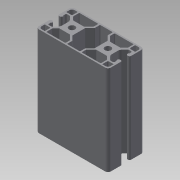
# Autodesk Inventor part: 40-4085-LITE
Saved by Autodesk Inventor 2013 (Build 170138000, 138)
## iProperties
Created: 2014-04-23
Part Number: 40-4085-LITE
Material: Generic
Document SubType Name: Modeling
Designer: Ross Bowman
Density: 1 g/cm^3
Engineer: Ross Bowman
Catalog Web Link: 8020.net
Vendor: 80/20 Inc.
Company: 80/20 Inc.
Author: Ross Bowman
Keywords: 80/20 , 8020 , T-Slot , Extrusion
Material: 6105-T5 Aluminum
Autodesk Inventor part; units mm, degrees
ref_plane "YZ Plane" through (0, 0, 0) normal (1, 0, 0) x (0, 1, 0)
ref_plane "XZ Plane" through (0, 0, 0) normal (0, 1, 0) x (-1, 0, 0)
ref_plane "XY Plane" through (0, 0, 0) normal (0, 0, 1) x (1, 0, 0)
sketch "Sketch1" plane through (0, 0, 0) normal (0, 0, 1) x (1, 0, 0)
  circle A0 centre (-20, 0) radius 3.3778
  circle A1 centre (20, 0) radius 3.3778
  arc A2 (-7.1746, -12.8345) -> (-7.435, -12.2058) centre (-8.0636, -12.8345) ccw
  line L0 (-12.0571, -7.5838) -> (-7.435, -12.2058)
  arc A3 (-12.3175, -6.9551) -> (-12.0571, -7.5838) centre (-11.4285, -6.9551) ccw
  line L1 (-12.3175, 7.0078) -> (-12.3175, -6.9551)
  arc A4 (-12.0943, 7.5465) -> (-12.3175, 7.0078) centre (-11.5556, 7.0078) ccw
  line L2 (-7.3343, 12.3066) -> (-12.0943, 7.5465)
  arc A5 (-7.3343, 12.3066) -> (-7.1111, 12.8453) centre (-7.873, 12.8453) ccw
  line L3 (-7.1111, 17.5873) -> (-7.1111, 12.8453)
  arc A6 (-6.3492, 18.3492) -> (-7.1111, 17.5873) centre (-6.3492, 17.5873) ccw
  line L4 (6.3492, 18.3492) -> (-6.3492, 18.3492)
  arc A7 (7.1111, 17.5873) -> (6.3492, 18.3492) centre (6.3492, 17.5873) ccw
  line L5 (7.1111, 12.8453) -> (7.1111, 17.5873)
  arc A8 (7.1111, 12.8453) -> (7.3343, 12.3066) centre (7.873, 12.8453) ccw
  line L6 (12.0943, 7.5465) -> (7.3343, 12.3066)
  arc A9 (12.3175, 7.0078) -> (12.0943, 7.5465) centre (11.5556, 7.0078) ccw
  line L7 (12.3175, -6.9551) -> (12.3175, 7.0078)
  arc A10 (12.0571, -7.5838) -> (12.3175, -6.9551) centre (11.4285, -6.9551) ccw
  line L8 (7.435, -12.2058) -> (12.0571, -7.5838)
  arc A11 (7.435, -12.2058) -> (7.1746, -12.8345) centre (8.0636, -12.8345) ccw
  line L9 (7.1746, -17.5873) -> (7.1746, -12.8345)
  arc A12 (6.4127, -18.3492) -> (7.1746, -17.5873) centre (6.4127, -17.5873) ccw
  line L10 (-6.4127, -18.3492) -> (6.4127, -18.3492)
  arc A13 (-7.1746, -17.5873) -> (-6.4127, -18.3492) centre (-6.4127, -17.5873) ccw
  line L11 (-7.1746, -12.8345) -> (-7.1746, -17.5873)
  arc A14 (9.239, -13.0955) -> (9.0159, -13.6343) centre (9.7778, -13.6343) ccw
  line L12 (14.4289, -7.9057) -> (9.239, -13.0955)
  arc A15 (14.9676, -7.6825) -> (14.4289, -7.9057) centre (14.9676, -8.4444) ccw
  line L13 (26.1099, -7.6825) -> (14.9676, -7.6825)
  arc A16 (26.6486, -7.9057) -> (26.1099, -7.6825) centre (26.1099, -8.4444) ccw
  line L14 (30.0626, -11.3196) -> (26.6486, -7.9057)
  arc A17 (30.2857, -11.8584) -> (30.0626, -11.3196) centre (29.5238, -11.8584) ccw
  line L15 (30.2857, -17.5873) -> (30.2857, -11.8584)
  arc A18 (29.5238, -18.3492) -> (30.2857, -17.5873) centre (29.5238, -17.5873) ccw
  line L16 (9.7778, -18.3492) -> (29.5238, -18.3492)
  arc A19 (9.0159, -17.5873) -> (9.7778, -18.3492) centre (9.7778, -17.5873) ccw
  line L17 (9.0159, -13.6343) -> (9.0159, -17.5873)
  arc A20 (-26.6486, 7.9057) -> (-26.1099, 7.6825) centre (-26.1099, 8.4444) ccw
  line L18 (-30.0626, 11.3196) -> (-26.6486, 7.9057)
  arc A21 (-30.2857, 11.8584) -> (-30.0626, 11.3196) centre (-29.5238, 11.8584) ccw
  line L19 (-30.2857, 17.5873) -> (-30.2857, 11.8584)
  arc A22 (-29.5238, 18.3492) -> (-30.2857, 17.5873) centre (-29.5238, 17.5873) ccw
  line L20 (-9.7778, 18.3492) -> (-29.5238, 18.3492)
  arc A23 (-9.0159, 17.5873) -> (-9.7778, 18.3492) centre (-9.7778, 17.5873) ccw
  line L21 (-9.0159, 13.6343) -> (-9.0159, 17.5873)
  arc A24 (-9.239, 13.0955) -> (-9.0159, 13.6343) centre (-9.7778, 13.6343) ccw
  line L22 (-14.4289, 7.9057) -> (-9.239, 13.0955)
  arc A25 (-14.9676, 7.6825) -> (-14.4289, 7.9057) centre (-14.9676, 8.4444) ccw
  line L23 (-26.1099, 7.6825) -> (-14.9676, 7.6825)
  arc A26 (-26.1099, -7.6825) -> (-26.6486, -7.9057) centre (-26.1099, -8.4444) ccw
  line L24 (-14.9676, -7.6825) -> (-26.1099, -7.6825)
  arc A27 (-14.4289, -7.9057) -> (-14.9676, -7.6825) centre (-14.9676, -8.4444) ccw
  line L25 (-9.239, -13.0955) -> (-14.4289, -7.9057)
  arc A28 (-9.0159, -13.6343) -> (-9.239, -13.0955) centre (-9.7778, -13.6343) ccw
  line L26 (-9.0159, -17.5873) -> (-9.0159, -13.6343)
  arc A29 (-9.7778, -18.3492) -> (-9.0159, -17.5873) centre (-9.7778, -17.5873) ccw
  line L27 (-29.5238, -18.3492) -> (-9.7778, -18.3492)
  arc A30 (-30.2857, -17.5873) -> (-29.5238, -18.3492) centre (-29.5238, -17.5873) ccw
  line L28 (-30.2857, -11.8584) -> (-30.2857, -17.5873)
  arc A31 (-30.0626, -11.3196) -> (-30.2857, -11.8584) centre (-29.5238, -11.8584) ccw
  line L29 (-26.6486, -7.9057) -> (-30.0626, -11.3196)
  arc A32 (9.7778, 18.3492) -> (9.0159, 17.5873) centre (9.7778, 17.5873) ccw
  line L30 (29.5238, 18.3492) -> (9.7778, 18.3492)
  arc A33 (30.2857, 17.5873) -> (29.5238, 18.3492) centre (29.5238, 17.5873) ccw
  line L31 (30.2857, 11.8584) -> (30.2857, 17.5873)
  arc A34 (30.0626, 11.3196) -> (30.2857, 11.8584) centre (29.5238, 11.8584) ccw
  line L32 (26.6486, 7.9057) -> (30.0626, 11.3196)
  arc A35 (26.1099, 7.6825) -> (26.6486, 7.9057) centre (26.1099, 8.4444) ccw
  line L33 (14.9676, 7.6825) -> (26.1099, 7.6825)
  arc A36 (14.4289, 7.9057) -> (14.9676, 7.6825) centre (14.9676, 8.4444) ccw
  line L34 (9.239, 13.0955) -> (14.4289, 7.9057)
  arc A37 (9.0159, 13.6343) -> (9.239, 13.0955) centre (9.7778, 13.6343) ccw
  line L35 (9.0159, 17.5873) -> (9.0159, 13.6343)
  arc A38 (32.3165, 18.3492) -> (31.9365, 17.9693) centre (32.3165, 17.9693) ccw
  line L36 (35.5555, 18.3492) -> (32.3165, 18.3492)
  arc A39 (38.3495, 15.5552) -> (35.5555, 18.3492) centre (35.5555, 15.5552) ccw
  line L37 (38.3495, 12.3165) -> (38.3495, 15.5552)
  arc A40 (37.9695, 11.9365) -> (38.3495, 12.3165) centre (37.9695, 12.3165) ccw
  line L38 (33.2063, 11.9365) -> (37.9695, 11.9365)
  arc A41 (31.9365, 13.2063) -> (33.2063, 11.9365) centre (33.2063, 13.2063) ccw
  line L39 (31.9365, 17.9693) -> (31.9365, 13.2063)
  arc A42 (35.5555, -18.3492) -> (38.3495, -15.5552) centre (35.5555, -15.5552) ccw
  line L40 (32.3165, -18.3492) -> (35.5555, -18.3492)
  arc A43 (31.9365, -17.9693) -> (32.3165, -18.3492) centre (32.3165, -17.9693) ccw
  line L41 (31.9365, -13.2063) -> (31.9365, -17.9693)
  arc A44 (33.2063, -11.9365) -> (31.9365, -13.2063) centre (33.2063, -13.2063) ccw
  line L42 (37.9695, -11.9365) -> (33.2063, -11.9365)
  arc A45 (38.3495, -12.3165) -> (37.9695, -11.9365) centre (37.9695, -12.3165) ccw
  line L43 (38.3495, -15.5552) -> (38.3495, -12.3165)
  arc A46 (-35.5555, 18.3492) -> (-38.3495, 15.5552) centre (-35.5555, 15.5552) ccw
  line L44 (-32.3165, 18.3492) -> (-35.5555, 18.3492)
  arc A47 (-31.9365, 17.9693) -> (-32.3165, 18.3492) centre (-32.3165, 17.9693) ccw
  line L45 (-31.9365, 13.2063) -> (-31.9365, 17.9693)
  arc A48 (-33.2063, 11.9365) -> (-31.9365, 13.2063) centre (-33.2063, 13.2063) ccw
  line L46 (-37.9695, 11.9365) -> (-33.2063, 11.9365)
  arc A49 (-38.3495, 12.3165) -> (-37.9695, 11.9365) centre (-37.9695, 12.3165) ccw
  line L47 (-38.3495, 15.5552) -> (-38.3495, 12.3165)
  arc A50 (-32.3165, -18.3492) -> (-31.9365, -17.9693) centre (-32.3165, -17.9693) ccw
  line L48 (-35.5555, -18.3492) -> (-32.3165, -18.3492)
  arc A51 (-38.3495, -15.5552) -> (-35.5555, -18.3492) centre (-35.5555, -15.5552) ccw
  line L49 (-38.3495, -12.3165) -> (-38.3495, -15.5552)
  arc A52 (-37.9695, -11.9365) -> (-38.3495, -12.3165) centre (-37.9695, -12.3165) ccw
  line L50 (-33.2063, -11.9365) -> (-37.9695, -11.9365)
  arc A53 (-31.9365, -13.2063) -> (-33.2063, -11.9365) centre (-33.2063, -13.2063) ccw
  line L51 (-31.9365, -17.9693) -> (-31.9365, -13.2063)
  arc A54 (35.4286, -10.2857) -> (36.6984, -9.0159) centre (35.4286, -9.0159) ccw
  line L52 (35.4286, -10.2857) -> (32.9885, -10.2857)
  arc A55 (32.3599, -10.0254) -> (32.9885, -10.2857) centre (32.9885, -9.3968) ccw
  line L53 (32.3599, -10.0254) -> (29.0736, -6.739)
  arc A56 (27.6825, -3.3808) -> (29.0736, -6.739) centre (32.4317, -3.3808) ccw
  line L54 (27.6825, -3.3808) -> (27.6825, 3.3808)
  arc A57 (29.0736, 6.739) -> (27.6825, 3.3808) centre (32.4317, 3.3808) ccw
  line L55 (29.0736, 6.739) -> (32.3599, 10.0254)
  arc A58 (32.9885, 10.2857) -> (32.3599, 10.0254) centre (32.9885, 9.3968) ccw
  line L56 (32.9885, 10.2857) -> (35.4286, 10.2857)
  arc A59 (36.6984, 9.0159) -> (35.4286, 10.2857) centre (35.4286, 9.0159) ccw
  line L57 (36.6984, 9.0159) -> (36.6984, 7.1685)
  arc A60 (36.3317, 6.7888) -> (36.6984, 7.1685) centre (36.3185, 7.1685) ccw
  line L58 (36.3317, 6.7888) -> (36.3032, 6.7878)
  arc A61 (36.3032, 6.7878) -> (35.9365, 6.4081) centre (36.3165, 6.4081) ccw
  line L59 (35.9365, 6.4081) -> (35.9365, 5.6381)
  arc A62 (35.9365, 5.6381) -> (37.5111, 4.0635) centre (37.5111, 5.6381) ccw
  line L60 (37.5111, 4.0635) -> (38.4254, 4.0635)
  arc A63 (38.4254, 4.0635) -> (40, 5.6381) centre (38.4254, 5.6381) ccw
  line L61 (40, 5.6381) -> (40, 16.8254)
  arc A64 (40, 16.8254) -> (36.8254, 20) centre (36.8254, 16.8254) ccw
  line L62 (36.8254, 20) -> (-36.8254, 20)
  arc A65 (-36.8254, 20) -> (-40, 16.8254) centre (-36.8254, 16.8254) ccw
  line L63 (-40, 16.8254) -> (-40, 5.6381)
  arc A66 (-40, 5.6381) -> (-38.4254, 4.0635) centre (-38.4254, 5.6381) ccw
  line L64 (-38.4254, 4.0635) -> (-37.5111, 4.0635)
  arc A67 (-37.5111, 4.0635) -> (-35.9365, 5.6381) centre (-37.5111, 5.6381) ccw
  line L65 (-35.9365, 5.6381) -> (-35.9365, 6.3446)
  arc A68 (-35.9365, 6.3446) -> (-36.3032, 6.7243) centre (-36.3165, 6.3446) ccw
  line L66 (-36.3032, 6.7243) -> (-36.3317, 6.7253)
  arc A69 (-36.6984, 7.105) -> (-36.3317, 6.7253) centre (-36.3185, 7.105) ccw
  line L67 (-36.6984, 7.105) -> (-36.6984, 9.0159)
  arc A70 (-35.4286, 10.2857) -> (-36.6984, 9.0159) centre (-35.4286, 9.0159) ccw
  line L68 (-35.4286, 10.2857) -> (-32.9885, 10.2857)
  arc A71 (-32.3599, 10.0254) -> (-32.9885, 10.2857) centre (-32.9885, 9.3968) ccw
  line L69 (-32.3599, 10.0254) -> (-29.0736, 6.739)
  arc A72 (-27.6825, 3.3808) -> (-29.0736, 6.739) centre (-32.4317, 3.3808) ccw
  line L70 (-27.6825, 3.3808) -> (-27.6825, -3.3808)
  arc A73 (-29.0736, -6.739) -> (-27.6825, -3.3808) centre (-32.4317, -3.3808) ccw
  line L71 (-29.0736, -6.739) -> (-32.3599, -10.0254)
  arc A74 (-32.9885, -10.2857) -> (-32.3599, -10.0254) centre (-32.9885, -9.3968) ccw
  line L72 (-32.9885, -10.2857) -> (-35.4286, -10.2857)
  arc A75 (-36.6984, -9.0159) -> (-35.4286, -10.2857) centre (-35.4286, -9.0159) ccw
  line L73 (-36.6984, -9.0159) -> (-36.6984, -7.105)
  arc A76 (-36.3317, -6.7253) -> (-36.6984, -7.105) centre (-36.3185, -7.105) ccw
  line L74 (-36.3317, -6.7253) -> (-36.3032, -6.7243)
  arc A77 (-36.3032, -6.7243) -> (-35.9365, -6.3446) centre (-36.3165, -6.3446) ccw
  line L75 (-35.9365, -6.3446) -> (-35.9365, -5.6381)
  arc A78 (-35.9365, -5.6381) -> (-37.5111, -4.0635) centre (-37.5111, -5.6381) ccw
  line L76 (-37.5111, -4.0635) -> (-38.4254, -4.0635)
  arc A79 (-38.4254, -4.0635) -> (-40, -5.6381) centre (-38.4254, -5.6381) ccw
  line L77 (-40, -5.6381) -> (-40, -16.8254)
  arc A80 (-40, -16.8254) -> (-36.8254, -20) centre (-36.8254, -16.8254) ccw
  line L78 (-36.8254, -20) -> (36.8254, -20)
  arc A81 (36.8254, -20) -> (40, -16.8254) centre (36.8254, -16.8254) ccw
  line L79 (40, -16.8254) -> (40, -5.6381)
  arc A82 (40, -5.6381) -> (38.4254, -4.0635) centre (38.4254, -5.6381) ccw
  line L80 (38.4254, -4.0635) -> (37.5111, -4.0635)
  arc A83 (37.5111, -4.0635) -> (35.9365, -5.6381) centre (37.5111, -5.6381) ccw
  line L81 (35.9365, -5.6381) -> (35.9365, -6.4081)
  arc A84 (35.9365, -6.4081) -> (36.3032, -6.7878) centre (36.3165, -6.4081) ccw
  line L82 (36.3032, -6.7878) -> (36.3317, -6.7888)
  arc A85 (36.6984, -7.1685) -> (36.3317, -6.7888) centre (36.3185, -7.1685) ccw
  line L83 (36.6984, -7.1685) -> (36.6984, -9.0159)
  point P0 (0, 0)
  constraints: 168 end point, 168 point on circle, 86 centre point
extrude "Extrusion1" add sketch "Sketch1" against normal blind 100
body "Solid1"
